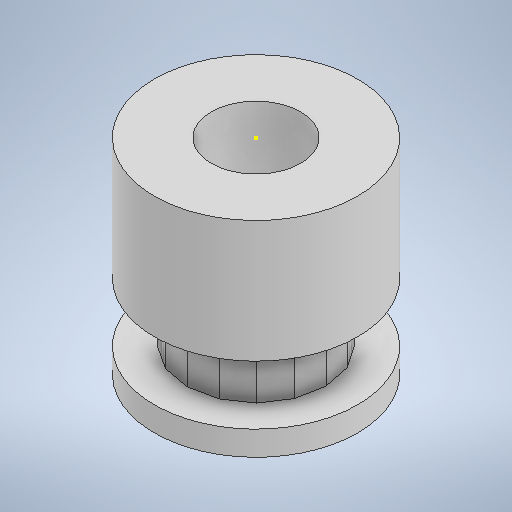
# Autodesk Inventor part: spool_long
Saved by Autodesk Inventor 2025.2 (Build 292293000, 293)
## iProperties
Created: 2024-12-25
Part Number: spool_long
Material: Ogólny
Document SubType Name: Modeling
Designer: Mos
Density: 1 g/cm^3
Appearance: Domyślna
Author: Mos
Autodesk Inventor part; units mm, degrees
ref_plane "YZ Plane" through (0, 0, 0) normal (1, 0, 0) x (0, 1, 0)
ref_plane "XZ Plane" through (0, 0, 0) normal (0, 1, 0) x (-1, 0, 0)
ref_plane "XY Plane" through (0, 0, 0) normal (0, 0, 1) x (1, 0, 0)
sketch "Szkic1" plane through (0, 0, 0) normal (0, 1, 0) x (-1, 0, 0)
  circle A0 centre (0, 0) radius 12.5
  dimension "d0" = 25
  constraints: 1 centre point, 1 coincident
  measures "d0" diameter of A0
extrude "Wyciągnięcie proste1" add sketch "Szkic1" along normal blind 3
sketch "Szkic7" plane through (0, 3, 0) normal (0, 1, 0) x (1, 0, 0)
  line L0 (6, 6.109) -> (7.8811, 3.3479)
  line L1 (7.8811, 3.3479) -> (8.5624, 0.0771)
  line L2 (8.5624, 0.0771) -> (7.9401, -3.2055)
  line L3 (7.9401, -3.2055) -> (6.109, -6)
  line L4 (6.109, -6) -> (3.3479, -7.8811)
  line L5 (3.3479, -7.8811) -> (0.0771, -8.5624)
  line L6 (0.0771, -8.5624) -> (-3.2055, -7.9401)
  line L7 (-3.2055, -7.9401) -> (-6, -6.109)
  line L8 (-6, -6.109) -> (-7.8811, -3.3479)
  line L9 (-7.8811, -3.3479) -> (-8.5624, -0.0771)
  line L10 (-8.5624, -0.0771) -> (-7.9401, 3.2055)
  line L11 (-7.9401, 3.2055) -> (-6.109, 6)
  line L12 (-6.109, 6) -> (-3.3479, 7.8811)
  line L13 (-3.3479, 7.8811) -> (-0.0771, 8.5624)
  line L14 (-0.0771, 8.5624) -> (3.2055, 7.9401)
  line L15 (3.2055, 7.9401) -> (6, 6.109)
  point P0 (0, 0)
  point P1 (0, 0)
  constraints: 32 end point, 1 coincident, 33 other
extrude "Wyciągnięcie proste6" add sketch "Szkic7" along normal blind 7.25
sketch "Szkic8" plane through (0, 10.25, 0) normal (0, 1, 0) x (1, 0, 0)
  circle A0 centre (0, 0) radius 12.5
  constraints: 1 centre point, 1 coincident
extrude "Wyciągnięcie proste7" add sketch "Szkic8" along normal blind 15
sketch "Szkic9" plane through (0, 25.25, 0) normal (0, 1, 0) x (1, 0, 0)
  circle A0 centre (0, 0) radius 5.5016
  constraints: 1 centre point, 1 coincident
extrude "Wyciągnięcie proste8" cut sketch "Szkic9" against normal blind 30
sketch "Szkic10" plane through (0, 25.25, 0) normal (0, 1, 0) x (1, 0, 0)
  point P0 (0, 0)
